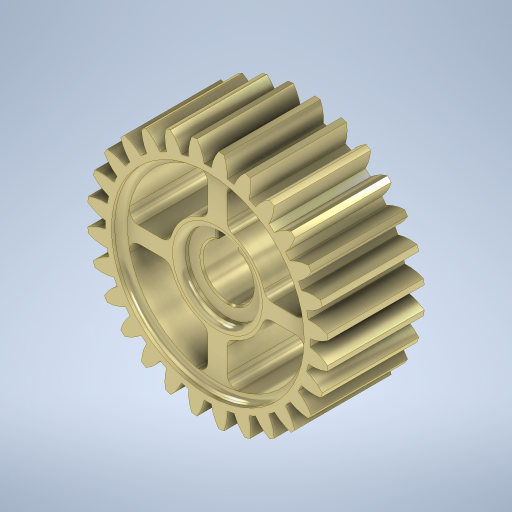
# Autodesk Inventor part: Engrenagem - Part 1
Saved by Autodesk Inventor 2023 (Build 270158030, 158C)
## iProperties
Created: 2022-07-18
Part Number: Engrenagem - Part 1
Material: Generic
Document SubType Name: Modeling
Designer: coqui
Density: 1 g/cm^3
Appearance: Gold - Metal
Author: coqui
Autodesk Inventor part; units mm, degrees
ref_plane "YZ Plane" through (0, 0, 0) normal (1, 0, 0) x (0, 1, 0)
ref_plane "XZ Plane" through (0, 0, 0) normal (0, 1, 0) x (-1, 0, 0)
ref_plane "XY Plane" through (0, 0, 0) normal (0, 0, 1) x (1, 0, 0)
sketch "Sketch1" plane through (0, 0, 0) normal (0, 0, 1) x (1, 0, 0)
  circle A0 centre (0, 0) radius 35 construction
  line L0 (-47.3463, 0) -> (52.5163, 0) construction
  line L1 (0, -48.5263) -> (0, 56.3118) construction
  arc A1 (-1.1092, 31.8557) -> (-3.3567, 37.3495) centre (-13.8522, 29.8491) ccw
  arc A2 (3.3567, 37.3495) -> (1.1092, 31.8557) centre (13.8522, 29.8491) ccw
  arc A3 (1.1092, 31.8557) -> (-1.1092, 31.8557) centre (0, 0) ccw
  arc A4 (-8.1699, 30.8102) -> (-11.5836, 35.6661) centre (-20.147, 26.0183) ccw
  arc A5 (-6.0072, 31.3038) -> (-8.1699, 30.8102) centre (0, 0) ccw
  arc A6 (-5.0385, 37.16) -> (-6.0072, 31.3038) centre (6.8629, 32.1831) ccw
  arc A7 (-14.821, 28.2197) -> (-19.2296, 32.1943) centre (-25.4315, 20.8828) ccw
  arc A8 (-12.8223, 29.1822) -> (-14.821, 28.2197) centre (0, 0) ccw
  arc A9 (-13.1811, 35.1071) -> (-12.8223, 29.1822) centre (-0.4706, 32.9034) ccw
  arc A10 (-20.7289, 24.2142) -> (-25.9114, 27.1081) centre (-29.4407, 14.7002) ccw
  arc A11 (-18.9945, 25.5973) -> (-20.7289, 24.2142) centre (0, 0) ccw
  arc A12 (-20.6627, 31.2938) -> (-18.9945, 25.5973) centre (-7.7805, 31.9737) ccw
  arc A13 (-25.5973, 18.9945) -> (-31.2938, 20.6627) centre (-31.9737, 7.7805) ccw
  arc A14 (-24.2142, 20.7289) -> (-25.5973, 18.9945) centre (0, 0) ccw
  arc A15 (-27.1081, 25.9114) -> (-24.2142, 20.7289) centre (-14.7002, 29.4407) ccw
  arc A16 (-29.1822, 12.8223) -> (-35.1071, 13.1811) centre (-32.9034, 0.4706) ccw
  arc A17 (-28.2197, 14.821) -> (-29.1822, 12.8223) centre (0, 0) ccw
  arc A18 (-32.1943, 19.2296) -> (-28.2197, 14.821) centre (-20.8828, 25.4315) ccw
  arc A19 (-31.3038, 6.0072) -> (-37.16, 5.0385) centre (-32.1831, -6.8629) ccw
  arc A20 (-30.8102, 8.1699) -> (-31.3038, 6.0072) centre (0, 0) ccw
  arc A21 (-35.6661, 11.5836) -> (-30.8102, 8.1699) centre (-26.0183, 20.147) ccw
  arc A22 (-31.8557, -1.1092) -> (-37.3495, -3.3567) centre (-29.8491, -13.8522) ccw
  arc A23 (-31.8557, 1.1092) -> (-31.8557, -1.1092) centre (0, 0) ccw
  arc A24 (-37.3495, 3.3567) -> (-31.8557, 1.1092) centre (-29.8491, 13.8522) ccw
  arc A25 (-30.8102, -8.1699) -> (-35.6661, -11.5836) centre (-26.0183, -20.147) ccw
  arc A26 (-31.3038, -6.0072) -> (-30.8102, -8.1699) centre (0, 0) ccw
  arc A27 (-37.16, -5.0385) -> (-31.3038, -6.0072) centre (-32.1831, 6.8629) ccw
  arc A28 (-28.2197, -14.821) -> (-32.1943, -19.2296) centre (-20.8828, -25.4315) ccw
  arc A29 (-29.1822, -12.8223) -> (-28.2197, -14.821) centre (0, 0) ccw
  arc A30 (-35.1071, -13.1811) -> (-29.1822, -12.8223) centre (-32.9034, -0.4706) ccw
  arc A31 (-24.2142, -20.7289) -> (-27.1081, -25.9114) centre (-14.7002, -29.4407) ccw
  arc A32 (-25.5973, -18.9945) -> (-24.2142, -20.7289) centre (0, 0) ccw
  arc A33 (-31.2938, -20.6627) -> (-25.5973, -18.9945) centre (-31.9737, -7.7805) ccw
  arc A34 (-18.9945, -25.5973) -> (-20.6627, -31.2938) centre (-7.7805, -31.9737) ccw
  arc A35 (-20.7289, -24.2142) -> (-18.9945, -25.5973) centre (0, 0) ccw
  arc A36 (-25.9114, -27.1081) -> (-20.7289, -24.2142) centre (-29.4407, -14.7002) ccw
  arc A37 (-12.8223, -29.1822) -> (-13.1811, -35.1071) centre (-0.4706, -32.9034) ccw
  arc A38 (-14.821, -28.2197) -> (-12.8223, -29.1822) centre (0, 0) ccw
  arc A39 (-19.2296, -32.1943) -> (-14.821, -28.2197) centre (-25.4315, -20.8828) ccw
  arc A40 (-6.0072, -31.3038) -> (-5.0385, -37.16) centre (6.8629, -32.1831) ccw
  arc A41 (-8.1699, -30.8102) -> (-6.0072, -31.3038) centre (0, 0) ccw
  arc A42 (-11.5836, -35.6661) -> (-8.1699, -30.8102) centre (-20.147, -26.0183) ccw
  arc A43 (1.1092, -31.8557) -> (3.3567, -37.3495) centre (13.8522, -29.8491) ccw
  arc A44 (-1.1092, -31.8557) -> (1.1092, -31.8557) centre (0, 0) ccw
  arc A45 (-3.3567, -37.3495) -> (-1.1092, -31.8557) centre (-13.8522, -29.8491) ccw
  arc A46 (8.1699, -30.8102) -> (11.5836, -35.6661) centre (20.147, -26.0183) ccw
  arc A47 (6.0072, -31.3038) -> (8.1699, -30.8102) centre (0, 0) ccw
  arc A48 (5.0385, -37.16) -> (6.0072, -31.3038) centre (-6.8629, -32.1831) ccw
  arc A49 (14.821, -28.2197) -> (19.2296, -32.1943) centre (25.4315, -20.8828) ccw
  arc A50 (12.8223, -29.1822) -> (14.821, -28.2197) centre (0, 0) ccw
  arc A51 (13.1811, -35.1071) -> (12.8223, -29.1822) centre (0.4706, -32.9034) ccw
  arc A52 (20.7289, -24.2142) -> (25.9114, -27.1081) centre (29.4407, -14.7002) ccw
  arc A53 (18.9945, -25.5973) -> (20.7289, -24.2142) centre (0, 0) ccw
  arc A54 (20.6627, -31.2938) -> (18.9945, -25.5973) centre (7.7805, -31.9737) ccw
  arc A55 (25.5973, -18.9945) -> (31.2938, -20.6627) centre (31.9737, -7.7805) ccw
  arc A56 (24.2142, -20.7289) -> (25.5973, -18.9945) centre (0, 0) ccw
  arc A57 (27.1081, -25.9114) -> (24.2142, -20.7289) centre (14.7002, -29.4407) ccw
  arc A58 (29.1822, -12.8223) -> (35.1071, -13.1811) centre (32.9034, -0.4706) ccw
  arc A59 (28.2197, -14.821) -> (29.1822, -12.8223) centre (0, 0) ccw
  arc A60 (32.1943, -19.2296) -> (28.2197, -14.821) centre (20.8828, -25.4315) ccw
  arc A61 (31.3038, -6.0072) -> (37.16, -5.0385) centre (32.1831, 6.8629) ccw
  arc A62 (30.8102, -8.1699) -> (31.3038, -6.0072) centre (0, 0) ccw
  arc A63 (35.6661, -11.5836) -> (30.8102, -8.1699) centre (26.0183, -20.147) ccw
  arc A64 (31.8557, 1.1092) -> (37.3495, 3.3567) centre (29.8491, 13.8522) ccw
  arc A65 (31.8557, -1.1092) -> (31.8557, 1.1092) centre (0, 0) ccw
  arc A66 (37.3495, -3.3567) -> (31.8557, -1.1092) centre (29.8491, -13.8522) ccw
  arc A67 (30.8102, 8.1699) -> (35.6661, 11.5836) centre (26.0183, 20.147) ccw
  arc A68 (31.3038, 6.0072) -> (30.8102, 8.1699) centre (0, 0) ccw
  arc A69 (37.16, 5.0385) -> (31.3038, 6.0072) centre (32.1831, -6.8629) ccw
  arc A70 (28.2197, 14.821) -> (32.1943, 19.2296) centre (20.8828, 25.4315) ccw
  arc A71 (29.1822, 12.8223) -> (28.2197, 14.821) centre (0, 0) ccw
  arc A72 (35.1071, 13.1811) -> (29.1822, 12.8223) centre (32.9034, 0.4706) ccw
  arc A73 (24.2142, 20.7289) -> (27.1081, 25.9114) centre (14.7002, 29.4407) ccw
  arc A74 (25.5973, 18.9945) -> (24.2142, 20.7289) centre (0, 0) ccw
  arc A75 (31.2938, 20.6627) -> (25.5973, 18.9945) centre (31.9737, 7.7805) ccw
  arc A76 (18.9945, 25.5973) -> (20.6627, 31.2938) centre (7.7805, 31.9737) ccw
  arc A77 (20.7289, 24.2142) -> (18.9945, 25.5973) centre (0, 0) ccw
  arc A78 (25.9114, 27.1081) -> (20.7289, 24.2142) centre (29.4407, 14.7002) ccw
  arc A79 (12.8223, 29.1822) -> (13.1811, 35.1071) centre (0.4706, 32.9034) ccw
  arc A80 (14.821, 28.2197) -> (12.8223, 29.1822) centre (0, 0) ccw
  arc A81 (19.2296, 32.1943) -> (14.821, 28.2197) centre (25.4315, 20.8828) ccw
  arc A82 (6.0072, 31.3038) -> (5.0385, 37.16) centre (-6.8629, 32.1831) ccw
  arc A83 (8.1699, 30.8102) -> (6.0072, 31.3038) centre (0, 0) ccw
  arc A84 (11.5836, 35.6661) -> (8.1699, 30.8102) centre (20.147, 26.0183) ccw
  arc A85 (-3.3567, 37.3495) -> (-5.0385, 37.16) centre (0, 0) ccw
  arc A86 (-11.5836, 35.6661) -> (-13.1811, 35.1071) centre (0, 0) ccw
  arc A87 (-19.2296, 32.1943) -> (-20.6627, 31.2938) centre (0, 0) ccw
  arc A88 (-25.9114, 27.1081) -> (-27.1081, 25.9114) centre (0, 0) ccw
  arc A89 (-31.2938, 20.6627) -> (-32.1943, 19.2296) centre (0, 0) ccw
  arc A90 (-35.1071, 13.1811) -> (-35.6661, 11.5836) centre (0, 0) ccw
  arc A91 (-37.16, 5.0385) -> (-37.3495, 3.3567) centre (0, 0) ccw
  arc A92 (-37.3495, -3.3567) -> (-37.16, -5.0385) centre (0, 0) ccw
  arc A93 (-35.6661, -11.5836) -> (-35.1071, -13.1811) centre (0, 0) ccw
  arc A94 (-32.1943, -19.2296) -> (-31.2938, -20.6627) centre (0, 0) ccw
  arc A95 (-27.1081, -25.9114) -> (-25.9114, -27.1081) centre (0, 0) ccw
  arc A96 (-20.6627, -31.2938) -> (-19.2296, -32.1943) centre (0, 0) ccw
  arc A97 (-13.1811, -35.1071) -> (-11.5836, -35.6661) centre (0, 0) ccw
  arc A98 (-5.0385, -37.16) -> (-3.3567, -37.3495) centre (0, 0) ccw
  arc A99 (3.3567, -37.3495) -> (5.0385, -37.16) centre (0, 0) ccw
  arc A100 (11.5836, -35.6661) -> (13.1811, -35.1071) centre (0, 0) ccw
  arc A101 (19.2296, -32.1943) -> (20.6627, -31.2938) centre (0, 0) ccw
  arc A102 (25.9114, -27.1081) -> (27.1081, -25.9114) centre (0, 0) ccw
  arc A103 (31.2938, -20.6627) -> (32.1943, -19.2296) centre (0, 0) ccw
  arc A104 (35.1071, -13.1811) -> (35.6661, -11.5836) centre (0, 0) ccw
  arc A105 (37.16, -5.0385) -> (37.3495, -3.3567) centre (0, 0) ccw
  arc A106 (37.3495, 3.3567) -> (37.16, 5.0385) centre (0, 0) ccw
  arc A107 (35.6661, 11.5836) -> (35.1071, 13.1811) centre (0, 0) ccw
  arc A108 (32.1943, 19.2296) -> (31.2938, 20.6627) centre (0, 0) ccw
  arc A109 (27.1081, 25.9114) -> (25.9114, 27.1081) centre (0, 0) ccw
  arc A110 (20.6627, 31.2938) -> (19.2296, 32.1943) centre (0, 0) ccw
  arc A111 (13.1811, 35.1071) -> (11.5836, 35.6661) centre (0, 0) ccw
  arc A112 (5.0385, 37.16) -> (3.3567, 37.3495) centre (0, 0) ccw
  line L2 (3, -34.8737) -> (3, -34.8712)
  line L3 (-34.9428, 2) -> (-34.9419, 2)
  arc A113 (-6.72, 27.1816) -> (-27.4343, 5.6) centre (0, 0) ccw
  arc A114 (-5, 14.1421) -> (-14.4097, 4.1667) centre (0, 0) ccw
  arc A115 (-27.1816, -6.72) -> (-6.72, -27.1816) centre (0, 0) ccw
  arc A116 (-14.1421, -5) -> (-5, -14.1421) centre (0, 0) ccw
  arc A117 (5, -14.1421) -> (14.1421, -5) centre (0, 0) ccw
  arc A118 (14.4097, 4.1667) -> (5, 14.1421) centre (0, 0) ccw
  line L4 (-3, -24.2693) -> (-3, -16.9706)
  line L5 (3, -24.2693) -> (3, -16.9706)
  line L6 (-3, 16.9706) -> (-3, 24.2693)
  line L7 (3, 16.9706) -> (3, 24.2693)
  line L8 (-24.4949, 2) -> (-17.2916, 2)
  line L9 (-24.2693, -3) -> (-16.9706, -3)
  line L10 (17.2916, 2) -> (24.4949, 2)
  line L11 (34.9419, 2) -> (34.9428, 2)
  line L12 (16.9706, -3) -> (24.2693, -3)
  line L13 (34.8712, -3) -> (34.8737, -3)
  arc A119 (-5, 14.1421) -> (-3, 16.9706) centre (-6, 16.9706) ccw
  arc A120 (-3, 24.2693) -> (-6.72, 27.1816) centre (-6, 24.2693) ccw
  arc A121 (-27.4343, 5.6) -> (-24.4949, 2) centre (-24.4949, 5) ccw
  arc A122 (-17.2916, 2) -> (-14.4097, 4.1667) centre (-17.2916, 5) ccw
  arc A123 (-24.2693, -3) -> (-27.1816, -6.72) centre (-24.2693, -6) ccw
  arc A124 (-14.1421, -5) -> (-16.9706, -3) centre (-16.9706, -6) ccw
  arc A125 (-6.72, -27.1816) -> (-3, -24.2693) centre (-6, -24.2693) ccw
  arc A126 (-3, -16.9706) -> (-5, -14.1421) centre (-6, -16.9706) ccw
  arc A127 (5, -14.1421) -> (3, -16.9706) centre (6, -16.9706) ccw
  arc A128 (3, -24.2693) -> (6.72, -27.1816) centre (6, -24.2693) ccw
  arc A129 (16.9706, -3) -> (14.1421, -5) centre (16.9706, -6) ccw
  arc A130 (14.4097, 4.1667) -> (17.2916, 2) centre (17.2916, 5) ccw
  arc A131 (3, 16.9706) -> (5, 14.1421) centre (6, 16.9706) ccw
  arc A132 (6.72, 27.1816) -> (3, 24.2693) centre (6, 24.2693) ccw
  arc A133 (6.72, -27.1816) -> (27.1816, -6.72) centre (0, 0) ccw
  arc A134 (27.4343, 5.6) -> (6.72, 27.1816) centre (0, 0) ccw
  arc A135 (27.1816, -6.72) -> (24.2693, -3) centre (24.2693, -6) ccw
  arc A136 (24.4949, 2) -> (27.4343, 5.6) centre (24.4949, 5) ccw
  arc A137 (-3, 7.4162) -> (3, 7.4162) centre (0, 0) ccw
  line L14 (-3, 10) -> (3, 10)
  line L15 (-3, 10) -> (-3, 7.4162)
  line L16 (3, 10) -> (3, 7.4162)
  point P0 (0, 39.078)
  point P1 (0, 37.338)
  point P2 (-5.609, 41.1377)
  point P3 (0, 39.882)
  point P4 (-3, -27.8388)
  point P5 (-3, 27.8388)
  point P6 (3, 27.8388)
  point P7 (3, 14.6969)
  point P8 (-3, 14.6969)
  point P9 (-27.9285, 2)
  point P10 (-27.8388, -3)
  point P11 (-14.8661, 2)
  point P12 (-14.6969, -3)
  point P13 (3, -27.8388)
  point P14 (-3, -14.6969)
  point P15 (3, -14.6969)
  point P16 (14.6969, -3)
  point P17 (14.8661, 2)
  point P18 (27.8388, -3)
  point P19 (27.9285, 2)
  dimension "d1" = 70
  dimension "d19" = 360
  dimension "d27" = 3
  dimension "d28" = 3
  dimension "d29" = 16
  dimension "d30" = 6
  dimension "d31" = 3
  dimension "d32" = 10
  constraints: 240 point on circle, 110 centre point, 34 end point, 30 tangent, 17 point on line, 14 equal radius, 12 parallel, 4 coincident, 4 vertical, 3 horizontal, 1 symmetric about line, 367 other
  measures "d1" diameter of A0
  measures "d27" radius of A119
  measures "d28" radius of A135
  measures "d29" diameter of A137
  measures "d30" distance of L14.start L14.end
  measures "d31" horizontal distance of L14.start point (0, 0)
  measures "d32" distance from line of point (0, 0) L14
extrude "Extrusion1" add sketch "Sketch1" along normal mid plane 30
sketch "Sketch3" plane through (0, 0, -15) normal (0, 0, -1) x (-1, 0, 0)
  circle A0 centre (0, 0) radius 30
  dimension "d37" = 60
  constraints: 1 centre point, 1 coincident
  measures "d37" diameter of A0
extrude "Extrusion2" cut sketch "Sketch3" against normal blind 3
mirror "Mirror1" about plane through (0, 0, 0) normal (0, 0, 1) of "Extrusion2"
fillet "Fillet1" radius 2 1 edges at (30, 0, -12)
fillet "Fillet2" radius 2 1 edges at (30, 0, 12)
sketch "Sketch4" plane through (0, 0, -12) normal (0, 0, -1) x (-1, 0, 0)
  circle A0 centre (0, 0) radius 12
  dimension "d42" = 24
  constraints: 1 centre point, 1 coincident
  measures "d42" diameter of A0
extrude "Extrusion3" cut sketch "Sketch4" against normal blind 3
mirror "Mirror2" about plane through (0, 0, 0) normal (0, 0, 1) of "Extrusion3"
chamfer "Chamfer1" distance 0.5 angle 45 8 edges at (-3, 8.7081, -9) (0, 10, -9) (3, 8.7081, -9) (0, -8, -9) (-3, 8.7081, 9) (0, 10, 9) (3, 8.7081, 9) (0, -8, 9)
fillet "Fillet4" radius 2 2 edges at (12, 0, -12) (12, 0, 12)
body "Solid1"
